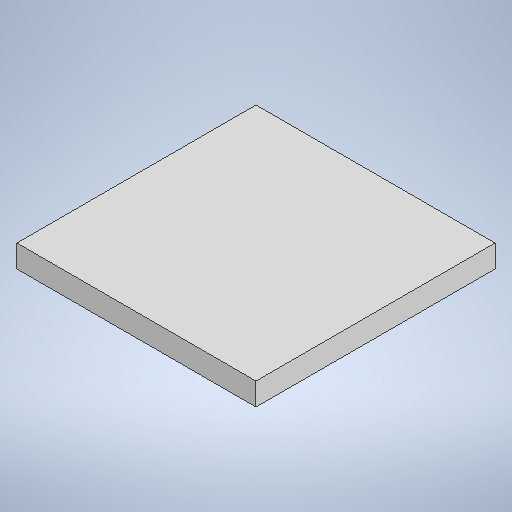
# Autodesk Inventor part: St3 16mm die stops X4
Saved by Autodesk Inventor 2025 (Build 290162010, 162A)
## iProperties
Created: 2024-06-21
Part Number: St3 16mm die stops X4
Material: Stainless Steel
Document SubType Name: Sheet Metal
Designer: admin
Density: 8 g/cm^3
Sheet Metal Rule: AISI304 2mm Die16
Appearance: Default
Flat Pattern Width: 8.5 cm
Flat Pattern Length: 8.5 cm
Flat Pattern Area: 72.25 cm^2
Sheet Metal Width: 85,000 mm
Sheet Metal Length: 85,000 mm
Sheet Metal Area: 7225,000 mm^2
Author: admin
Autodesk Inventor part; units mm, degrees
ref_plane "YZ Plane" through (0, 0, 0) normal (1, 0, 0) x (0, 1, 0)
ref_plane "XZ Plane" through (0, 0, 0) normal (0, 1, 0) x (-1, 0, 0)
ref_plane "XY Plane" through (0, 0, 0) normal (0, 0, 1) x (1, 0, 0)
sketch "Sketch1" plane through (0, 0, 0) normal (0, 0, 1) x (1, 0, 0)
  line L0 (-42.5, 85) -> (42.5, 85)
  line L1 (42.5, 85) -> (42.5, 0)
  line L2 (42.5, 0) -> (-42.5, 0)
  line L3 (-42.5, 0) -> (-42.5, 85)
  point P0 (0, 0)
  point P1 (0, 0)
  dimension "d0" = 85
  dimension "d4" = 85
  measures "d0" distance of L1.end L2.end
  measures "d4" distance of L2.end L0.start
extrude "Plate1" add sketch "Sketch1" along normal blind 8
equation "\"d4\" = d0"
equation "\"d10\" = Thickness"
equation "\"BendReliefWidth\" = Thickness"
equation "\"BendReliefDepth\" = 0.5 * Thickness"
equation "\"CornerReliefSize\" = 4 * Thickness"
equation "\"MinimumRemnant\" = 2 * Thickness"
equation "\"TransitionRadius\" = BendRadius"
equation "\"JacobiRadiusSize\" = BendRadius"
equation "\"GapSize\" = Thickness"
equation "\"Thickness\" = 8"
equation "\"BendRadius\" = 2.75"
body "Solid1"
